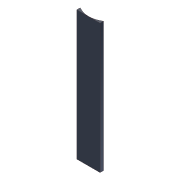
# Autodesk Inventor part: epoxy_under-battery
Saved by Autodesk Inventor 2014 SP1 (Build 180222100, 222)
## iProperties
Created: 2013-07-10
Part Number: epoxy_under-battery
Document SubType Name: Modeling
Designer: Robert Davis
Density: 1 g/cm^3
Material: Generic
Appearance: Default
Author: Robert Davis
Autodesk Inventor part; units mm, degrees
ref_plane "YZ Plane" through (0, 0, 0) normal (1, 0, 0) x (0, 1, 0)
ref_plane "XZ Plane" through (0, 0, 0) normal (0, 1, 0) x (-1, 0, 0)
ref_plane "XY Plane" through (0, 0, 0) normal (0, 0, 1) x (1, 0, 0)
sketch "Sketch1" plane through (0, 0, 0) normal (0, 0, 1) x (1, 0, 0)
  line L0 (4.5, 1.3479) -> (4.5, 0)
  line L1 (4.5, 0) -> (-4.5, 0)
  line L2 (-4.5, 0) -> (-4.5, 1.3479)
  arc A0 (-4.5, 1.3479) -> (4.5, 1.3479) centre (0, 8.5) ccw
  point P0 (0, 0)
  point P1 (0, 0)
  point P2 (0, 0.05)
  dimension "d0" = 9
  dimension "d1" = 8.45
  dimension "d2" = 8.5
  constraints: 6 end point, 3 point on circle, 2 vertical, 1 centre point, 1 coincident, 1 horizontal, 1 midpoint, 1 vertical alignment
  measures "d0" distance of L2.end L0.start
  measures "d1" radius of A0
  measures "d2" distance from line of L1 A0.centre
extrude "Extrusion1" add sketch "Sketch1" along normal mid plane 50
body "Solid1"
